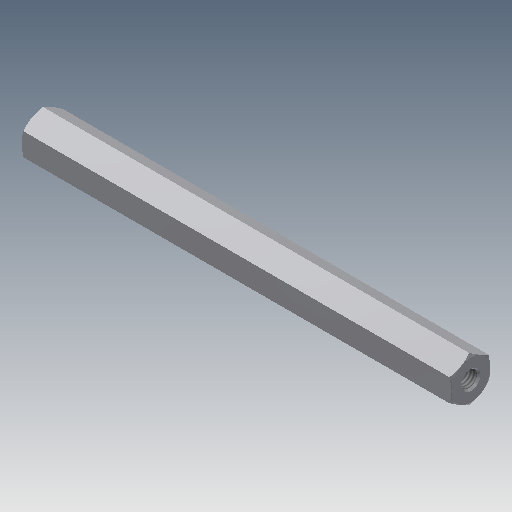
# Autodesk Inventor part: ALSFB6-66
Saved by Autodesk Inventor 2017.3 (Build 213256000, 256)
## iProperties
Category: PARTsolutions
Company: MISUMI
Created: 2016-05-23
Part Number: ALSFB6-66
Catalog Web Link: www.cadenas.de
Description: NLSFB, LSFB, PLSFB, BLSFB, SLSBFA, ALSFB-Hex Posts - Both Ends Tapped - L Dimension Configurable -
Vendor: MISUMI
Document SubType Name: Modeling
Designer: psAdmin
Manufacturer: MISUMI
Mass: 5.53172 g
Surface Area: 15.5851 cm^2
Volume: 1.97561 cm^3
Density: 2.8 g/cm^3
Material: アルミニウム 2014-T4
Appearance: サテン
PSOL_IDENT_0: {$CADENAS_DATA\23d-libs\misumi\metric\19_posts_stands\lsfb.prj},208 {VTYP=3D},{NB=ALSFB6-66},{LINA=A
PSOL_IDENT_1: LSFB6-66},{NN=NLSFB, LSFB, PLSFB, BLSFB, SLSBFA, ALSFB},{DATE=27.01.2016 00:40:47},{GEOMDATE=27.01.2
PSOL_IDENT_2: 016 00:40:47},{VERSION=},{LINEID=220},{LINESUBID=-1},{WBVAR=MAT,ST,ALT1,L}  {NB=ALSFB6-66},{LINA=ALS
PSOL_IDENT_3: FB6-66},{KT=DUMMY},{PN=ALSFB6-66},{TYPE=ALSFB},{MAT=2011},{MATALG='LCS','Low Carbon Steel', '304', '
PSOL_IDENT_4: SUS304','2011', '2011 Aluminum Alloy'},{ST=CA},{STALG= 'CA','Clear Anodizing' },{B=6},{ALT1=},{L=66.
PSOL_IDENT_5: 0},{LALG=[8:100/0.5]},{M=3},{MMAX=3},{C=6.9},{NAV=3},{MPITCH=0.5},{M3D1=6},{M3D2=9}
NN: NLSFB, LSFB, PLSFB, BLSFB, SLSBFA, ALSFB
NT: Hex Posts - Both Ends Tapped - L Dimension Configurable -
NB: ALSFB6-66
NBSYN: $PN.
LINA: ALSFB6-66
PN: ALSFB6-66
MAT: 2011 Aluminum Alloy
ST: Clear Anodize
B: 6
ALT1: w/o LKC (L Dimension Tolerance)
L: 66.0
M: 3
C: 6.9
SUPPLIER: MISUMI
ARTICLENO: ALSFB6-66
BOMINFO: ALSFB6-66
CREATOR: CADENAS GmbH
Title: ALSFB6-66
Author: Cadenas PARTsolutions
Comments: Hex Posts - Both Ends Tapped - L Dimension Configurable -
Autodesk Inventor part; units mm, degrees
sketch "Sketch_1" plane through (0, 0, 0) normal (0, 0, 1) x (1, 0, 0)
  line L0 (66, 0) -> (0, 0)
  line L1 (0, 0) -> (0, 3)
  line L2 (0, 3) -> (2.2517, 6.9)
  line L3 (2.2517, 6.9) -> (63.7483, 6.9)
  line L4 (63.7483, 6.9) -> (66, 3)
  line L5 (66, 3) -> (66, 0)
  line L6 (66, 0) -> (0, 0)
  constraints: 14 end point
revolve "Revolution1" add sketch "Sketch_1" angle 360 about axis through (66, 0, 0) along (1, 0, 0)
sketch "Sketch_2" plane through (0, 0, 0) normal (1, 0, 0) x (0, 1, 0)
  line L0 (6.9, 6.9) -> (-6.9, 6.9)
  line L1 (-6.9, 6.9) -> (-6.9, -6.9)
  line L2 (-6.9, -6.9) -> (6.9, -6.9)
  line L3 (6.9, -6.9) -> (6.9, 6.9)
  line L4 (1.7321, 3) -> (-1.7321, 3)
  line L5 (-1.7321, 3) -> (-3.4641, 0)
  line L6 (-3.4641, 0) -> (-1.7321, -3)
  line L7 (-1.7321, -3) -> (1.7321, -3)
  line L8 (1.7321, -3) -> (3.4641, 0)
  line L9 (3.4641, 0) -> (1.7321, 3)
  constraints: 20 end point
extrude "Extrusion1" cut sketch "Sketch_2" along normal blind 66
sketch "Sketch3" plane through (0, 0, 0) normal (-1, 0, 0) x (0, 0, 1)
  point P0 (0, 0)
hole "Hole1" at (0, 0, 0) direction (1, 0, 0) diameter 2.459 depth 8.2901 tip angle 120 countersink diameter 3 countersink angle 90 thread size "M3x0.5" class "6H" standard "ISO Metric profile"
sketch "Sketch4" plane through (66, 0, 0) normal (1, 0, 0) x (0, 0, -1)
  point P0 (0, 0)
hole "Hole2" at (66, 0, 0) direction (-1, 0, 0) diameter 2.459 depth 8.2901 tip angle 120 countersink diameter 3 countersink angle 90 thread size "M3x0.5" class "6H" standard "ISO Metric profile"
ref_plane "C2_XY" through (0, 0, 0) normal (1, 0, 0) x (0, 0, -1)
ref_plane "C2_YZ" through (0, 0, 0) normal (0, 0, -1) x (0, 1, 0)
ref_plane "C2_ZX" through (0, 0, 0) normal (0, 1, 0) x (1, 0, 0)
body "Solid1"
